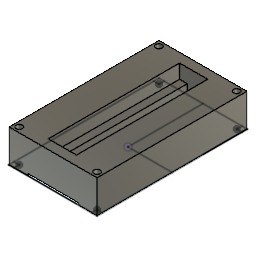
470nm_laser_mount (Autodesk Fusion 360 design; units mm, degrees)
Autodesk Fusion 360 part; units mm, degrees
note: some values were not read from the file. Set by a fixed rule: the direction of a hole.
sketch "Sketch1" plane through (0, 0, 0) normal (0, 0, 1) x (1, 0, 0)
  line L0 (-23.5, 40) -> (23.5, 40)
  line L1 (23.5, 40) -> (23.5, -40)
  line L2 (23.5, -40) -> (-23.5, -40)
  line L3 (-23.5, -40) -> (-23.5, 40)
  line L4 (0, 40) -> (0, 0)
  line L5 (0, 0) -> (23.5, 0)
  line L6 (-20.75, 37.25) -> (-23.5, 37.25)
  line L7 (-20.75, -37.25) -> (-23.5, -37.25)
  line L8 (20.75, -37.25) -> (23.5, -37.25)
  line L9 (20.75, 37.25) -> (23.5, 37.25)
  line L10 (-20.75, 37.25) -> (-20.75, 40)
  line L11 (20.75, 37.25) -> (20.75, 40)
  line L12 (20.75, -37.25) -> (20.75, -40)
  line L13 (-20.75, -37.25) -> (-20.75, -40)
  point P0 (-20.75, 37.25)
  point P1 (20.75, 37.25)
  point P2 (20.75, -37.25)
  point P3 (-20.75, -37.25)
  dimension "d2" = 47
  dimension "d3" = 80
  dimension "d4" = 2.75
  constraint horizontal L0
  constraint vertical L1
  constraint horizontal L2
  constraint vertical L3
  constraint midpoint L0 L4.start
  constraint coincident L4.end L5.start
  constraint perpendicular L0 L4
  constraint midpoint L1 L5.end
  constraint perpendicular L1 L5
  constraint coincident P0 L6.start
  constraint coincident L3 L6.end
  constraint perpendicular L3 L6
  constraint coincident P3 L7.start
  constraint coincident L3 L7.end
  constraint perpendicular L3 L7
  constraint coincident P2 L8.start
  constraint coincident L1 L8.end
  constraint perpendicular L1 L8
  constraint coincident P1 L9.start
  constraint coincident L1 L9.end
  constraint perpendicular L1 L9
  constraint perpendicular L6 L10
  constraint perpendicular L9 L11
  constraint coincident L2 L12.end
  constraint perpendicular L2 L12
  constraint coincident L2 L13.end
  constraint perpendicular L2 L13
  constraint equal L6 L10
  constraint equal L10 L11
  constraint equal L9 L11
  constraint equal L7 L13
  constraint equal L8 L12
  constraint equal L7 L10
  constraint equal L10 L12
  constraint coincident L0 L11.end
  constraint coincident L0 L10.end
  measures "d2" distance of L0.start L0.end
  measures "d3" distance of L0.end L1.end
  measures "d4" distance of P0 L10.end
extrude "Extrude1" add sketch "Sketch1" along normal blind 17.5
hole "Hole1" at (-20.75, 37.25, 0) at (20.75, 37.25, 0) at (-20.75, -37.25, 0) at (20.75, -37.25, 0) direction (0, 0, 1) diameter 3.3 end through all
sketch "Sketch2" plane through (0, 0, 17.5) normal (0, 0, 1) x (-1, 0, 0)
  circle A0 centre (20.75, 37.25) radius 1.65
  circle A1 centre (20.75, -37.25) radius 1.65
  circle A2 centre (-20.75, -37.25) radius 1.65
  circle A3 centre (-20.75, 37.25) radius 1.65
  line L0 (23.5, 40) -> (-23.5, 40)
  line L1 (-23.5, 40) -> (-23.5, -40)
  line L2 (-23.5, -40) -> (23.5, -40)
  line L3 (23.5, -40) -> (23.5, 40)
  line L4 (0, 0) -> (-7.5, 0)
  line L5 (0, 0) -> (0, -35)
  line L6 (7.5, -35) -> (-7.5, -35)
  line L7 (-7.5, -35) -> (-7.5, 35)
  line L8 (-7.5, 35) -> (7.5, 35)
  line L9 (7.5, 35) -> (7.5, -35)
  dimension "d12" = 15
  dimension "d13" = 70
  constraint coincident L4.start L5.start
  constraint horizontal L4
  constraint perpendicular L4 L5
  constraint horizontal L6
  constraint vertical L7
  constraint horizontal L8
  constraint vertical L9
  constraint coincident L4.end L7
  constraint midpoint L5.end L6
  constraint midpoint L4.end L7
  measures "d12" distance of L6.start L6.end
  measures "d13" distance of L6.end L7.end
extrude "Extrude2" cut sketch "Sketch2" against normal blind 7.5 contours L4 L5 L6 L7 | L4 L5 L6 L7 L8 L9
sketch "Sketch3" plane through (0, 0, 10) normal (0, 0, 1) x (-1, 0, 0)
  line L0 (7.5, 35) -> (-7.5, 35)
  line L1 (-7.5, 35) -> (-7.5, -35)
  line L2 (-7.5, -35) -> (7.5, -35)
  line L3 (7.5, -35) -> (7.5, 35)
  line L4 (0, 0) -> (0, -35)
  line L5 (0, 0) -> (-3.375, 0)
  line L6 (3.375, -35) -> (-3.375, -35)
  line L7 (-3.375, -35) -> (-3.375, 35)
  line L8 (-3.375, 35) -> (3.375, 35)
  line L9 (3.375, 35) -> (3.375, -35)
  dimension "d16" = 70
  dimension "d17" = 6.75
  constraint coincident L4.start L5.start
  constraint vertical L4
  constraint perpendicular L4 L5
  constraint horizontal L6
  constraint vertical L7
  constraint horizontal L8
  constraint vertical L9
  constraint midpoint L5.end L7
  constraint midpoint L4.end L6
  measures "d16" distance of L6.end L7.end
  measures "d17" distance of L6.start L6.end
extrude "Extrude3" cut sketch "Sketch3" against normal through all contours L0 L2 L4 L5 L6 L7 L8 L9 | L2 L4 L5 L6 L7
sketch "Sketch4" plane through (0, 0, 0) normal (0, 0, 1) x (1, 0, 0)
  line L0 (0, 0) -> (13.3476, 0)
  line L1 (0, 0) -> (0, -40)
  line L2 (-13.3476, -40) -> (13.3476, -40)
  line L3 (13.3476, -40) -> (13.3476, 40)
  line L4 (13.3476, 40) -> (-13.3476, 40)
  line L5 (-13.3476, 40) -> (-13.3476, -40)
  constraint coincident L0.start L1.start
  constraint horizontal L0
  constraint perpendicular L0 L1
  constraint horizontal L2
  constraint vertical L3
  constraint horizontal L4
  constraint vertical L5
  constraint midpoint L0.end L3
  constraint midpoint L1.end L2
extrude "Extrude4" cut sketch "Sketch4" along normal blind 1
